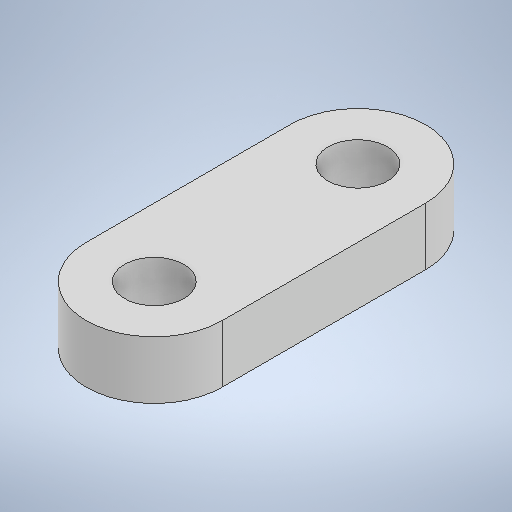
# Autodesk Inventor part: Direccion,2pero2.0
Saved by Autodesk Inventor 2025.2 (Build 292293000, 293)
## iProperties
Created: 2025-03-24
Part Number: Direccion,2pero2.0
Material: Genérico
Document SubType Name: Modeling
Designer: Gabi
Density: 1 g/cm^3
Appearance: Valor por defecto
Author: Gabi
Autodesk Inventor part; units mm, degrees
ref_plane "YZ Plane" through (0, 0, 0) normal (1, 0, 0) x (0, 1, 0)
ref_plane "XZ Plane" through (0, 0, 0) normal (0, 1, 0) x (-1, 0, 0)
ref_plane "XY Plane" through (0, 0, 0) normal (0, 0, 1) x (1, 0, 0)
sketch "Boceto1" plane through (0, 0, 0) normal (0, 1, 0) x (-1, 0, 0)
  circle A0 centre (0, 0) radius 1.75
  arc A1 (4, 0) -> (-4, 0) centre (0, 0) ccw
  line L0 (4, 0) -> (4, -12)
  line L1 (0, 0) -> (0, -1.75)
  line L2 (4, 0) -> (4, -6)
  line L3 (4, -6) -> (0, -6)
  line L4 (-4, 0) -> (-4, -12)
  circle A2 centre (0, -12) radius 1.75
  arc A3 (-4, -12) -> (4, -12) centre (0, -12) ccw
  dimension "d0" = 3.5
  dimension "d1" = 8
  dimension "d2" = 12
  dimension "d3" = 6
  constraints: 10 end point, 4 point on circle, 3 centre point, 3 coincident, 3 symmetric about line, 2 vertical, 1 midpoint, 1 perpendicular, 1 point on line, 1 tangent, 1 vertical alignment, 3 other
  measures "d1" diameter of A1
  measures "d2" distance of L0.start L0.end
  measures "d3" distance of L0.start L2.end
extrude "Extrusión1" add sketch "Boceto1" along normal blind 3.4
